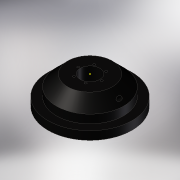
# Autodesk Inventor part: Part1
Saved by Autodesk Inventor 2021 (Build 250183000, 183)
## iProperties
Created: 2022-08-15
Part Number: Part1
Material: Stainless Steel
Document SubType Name: Sheet Metal
Designer: pc
Density: 8 g/cm^3
Sheet Metal Rule: Default_mm
Appearance: Stainless - Brushed
Mass: 3185.1 g
Surface Area: 658.474 cm^2
Volume: 398.137 cm^3
Author: pc
Autodesk Inventor part; units mm, degrees
ref_plane "XZ Plane" through (0, 0, 0) normal (0, 1, 0) x (-1, 0, 0)
sketch "Sketch1" plane through (0, 0, 0) normal (0, 0, 1) x (1, 0, 0)
  line L0 (0, 0) -> (0, 66)
  line L1 (75, -0.1929) -> (75, 14.8071)
  line L2 (-21.5975, 0) -> (0, 0)
  line L3 (46.9201, 0) -> (53.1744, 0)
  line L4 (75, 14.8071) -> (60, 14.8071)
  line L5 (60, 14.8071) -> (60, 34.8071)
  line L6 (0, 33.8071) -> (0, 49.8071)
  line L7 (0, 49.8071) -> (35, 49.8071)
  line L8 (46.9201, 9.8071) -> (40, 9.8071)
  line L9 (40, 9.8071) -> (40, 33.8071)
  line L10 (60, 34.8071) -> (60, 49.8071)
  line L11 (60, 49.8071) -> (35, 49.8071)
  line L12 (46.9201, 9.8071) -> (50, 9.8071)
  line L13 (50, 9.8071) -> (50, -0.1929)
  line L14 (50, -0.1929) -> (75, -0.1929)
  line L15 (0, 33.8071) -> (0, 9.8071)
  line L16 (0, 9.8071) -> (20, 9.8071)
  line L17 (20, 9.8071) -> (20, 33.8071)
  line L18 (20, 33.8071) -> (40, 33.8071)
  dimension "d0" = 66
  dimension "d2" = 150
  dimension "d4" = 15
  dimension "d5" = 20
  dimension "d15" = 35
  dimension "d16" = 70
  dimension "d84" = 100
  dimension "d92" = 50
  dimension "d132" = 15
  dimension "d134" = 10
  dimension "d136" = 40
  dimension "d137" = 20
  constraints: 38 end point, 7 perpendicular, 6 horizontal, 5 vertical, 1 point on line
  measures "d0" distance of L0.start L0.end
  measures "d2" diameter of L1 L0
  measures "d4" distance of L1.end L4.end
  measures "d5" distance of L4.end L5.end
  measures "d15" distance of L6.end L7.end
  measures "d16" diameter of L7.end L0
  measures "d84" diameter of L13 L0
  measures "d92" distance from line of L13.end L7
  measures "d132" distance of L1.start L1.end
  measures "d134" distance from line of L13.end L8
  measures "d136" diameter of L16.end L0
  measures "d137" distance between parallel lines of L5 L9
revolve "Revolution1" add sketch "Sketch1" angle 360 about axis through (0, 0, 0) along (0, 1, 0)
chamfer "Chamfer1" distance 20 angle 45 1 edges at (-60, 49.8071, 0)
ref_plane "Work Plane1" through (60, 0, 0) normal (1, 0, 0) x (0, 1, 0)
sketch "Sketch10" plane through (0, 49.8071, 0) normal (0, 1, 0) x (1, 0, 0)
  circle A0 centre (0, 0) radius 16
  dimension "d54" = 32
  constraints: 1 centre point, 1 coincident
  measures "d54" diameter of A0
hole "Hole2" at (0, 49.8071, 0) direction (0, -1, 0) diameter 35 end through all
ref_plane "Work Plane2" through (60, 0, 0) normal (1, 0, 0) x (0, 1, 0)
sketch "Sketch14" plane through (60, 0, 0) normal (1, 0, 0) x (0, 1, 0)
  circle A0 centre (45.5775, 0) radius 5
  point P0 (0, 0)
  dimension "d89" = 10
  constraints: 1 centre point
  measures "d89" diameter of A0
sketch "Sketch15" plane through (0, 0, 0) normal (0, 0, 1) x (1, 0, 0)
  line L0 (59.908, 45.3055) -> (36.1068, 21.3737)
  point P0 (0, 0)
  constraints: 2 end point
sweep "Sweep4" cut profiles "Sketch14" path "Sketch15"
sketch "Sketch18" plane through (0, 49.8071, 0) normal (0, 1, 0) x (1, 0, 0)
  point P0 (0, 0)
sketch "Sketch19" plane through (0, 49.8071, 0) normal (0, 1, 0) x (1, 0, 0)
  circle A0 centre (-21, 0) radius 2
  circle A1 centre (-10.5, -18.1865) radius 2
  circle A2 centre (10.5, -18.1865) radius 2
  circle A3 centre (21, 0) radius 2
  circle A4 centre (10.5, 18.1865) radius 2
  circle A5 centre (-10.5, 18.1865) radius 2
  point P0 (0, 0)
  dimension "d144" = 4
  dimension "d145" = 21
  dimension "d148" = 360
  constraints: 6 centre point, 13 other
  measures "d144" diameter of A0
  measures "d145" distance of A0.centre point (0, 0)
hole "Hole5" at (-21, 49.8071, 0) at (-10.5, 49.8071, -18.1865) at (21, 49.8071, 0) at (10.5, 49.8071, 18.1865) at (-10.5, 49.8071, 18.1865) at (10.5, 49.8071, -18.1865) direction (0, -1, 0) diameter 4 depth 5 tip angle 118
thread "Thread21"
thread "Thread22"
thread "Thread23"
thread "Thread24"
thread "Thread25"
thread "Thread26"
equation "\"d60\" = Thickness"
equation "\"BendRadius\" = Thickness"
equation "\"BendReliefWidth\" = Thickness"
equation "\"BendReliefDepth\" = 0.5 * Thickness"
equation "\"CornerReliefSize\" = 4 * Thickness"
equation "\"MinimumRemnant\" = 2 * Thickness"
equation "\"TransitionRadius\" = BendRadius"
equation "\"JacobiRadiusSize\" = BendRadius"
equation "\"GapSize\" = Thickness"
equation "\"Thickness\" = 0.5"
body "Solid1"
